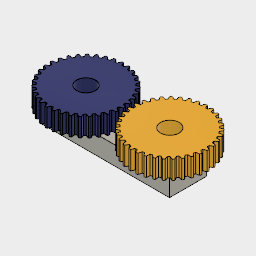
C04-W3-PE-01 (Autodesk Fusion 360 design; units mm, degrees)
Autodesk Fusion 360 part; units mm, degrees
sketch "Sketch1" plane through (0, 0, 0) normal (0, 1, 0) x (1, 0, 0) in component "Base Plate"
  line L0 (-87.5, 25) -> (87.5, 25)
  line L1 (87.5, 25) -> (87.5, -25)
  line L2 (87.5, -25) -> (-87.5, -25)
  line L3 (-87.5, -25) -> (-87.5, 25)
  line L4 (-87.5, 25) -> (87.5, -25) construction
  line L5 (87.5, 25) -> (-87.5, -25) construction
  circle A0 centre (-50, 0) radius 12.5
  circle A1 centre (50, 0) radius 12.5
  dimension "d1" = 175
  dimension "d2" = 50
  dimension "d3" = 25
  dimension "d4" = 50
  dimension "d5" = 50
  measures "d1" distance of L1.end L2.end
  measures "d2" distance of L0.end L1.end
  measures "d3" diameter of A1
  measures "d4" distance of origin A0.centre
  measures "d5" distance of origin A1.centre
extrude "Extrude1" add sketch "Sketch1" along normal blind 25 makes body 1 in component "Base Plate"
sketch "Sketch1 (2)" plane through (0, 25, 0) normal (0, 1, 0) x (-1, 0, 0) in component "Gear 1"
  circle A0 centre (-50, 0) radius 12.5
  circle A1 centre (50, 0) radius 12.5
  line L0 (87.5, 25) -> (-87.5, 25)
  line L1 (-87.5, 25) -> (-87.5, -25)
  line L2 (-87.5, -25) -> (87.5, -25)
  line L3 (87.5, -25) -> (87.5, 25)
  circle A2 centre (50, 0) radius 12.5
  circle A3 centre (50, 0) radius 47.5
  dimension "d19" = 95
  measures "d19" diameter of A3
extrude "Extrude1'" add sketch "Sketch1 (2)" along normal blind 25 separate body contours L0 L2 L3 A3 | L0 L2 L3 A3 makes body 2 in component "Gear 1"
sketch "Sketch2" plane through (0, 50, 0) normal (0, 1, 0) x (-1, 0, 0) in component "Gear 1"
  circle A0 centre (50, 0) radius 12.5
  circle A1 centre (50, 0) radius 47.5
  line L0 (0, 0) -> (-2, 0) construction
  arc A2 (-1.6663, 1.375) -> (-1.6663, -1.375) centre (1, 0) ccw
  line L1 (-1.6663, -1.375) -> (2.5901, -2.9242)
  line L2 (-1.6663, 1.375) -> (2.5901, 2.9242)
  dimension "d10" = 2
  dimension "d11" = 3
  dimension "d12" = 2.75
  dimension "d13" = 20
  dimension "d14" = 20
  measures "d10" distance of L0.start L0.end
  measures "d11" radius of A2
  measures "d12" distance of A2.end A2.start
  measures "d13" angle of L0 L1
  measures "d14" angle of L0 L2
extrude "Extrude2" add sketch "Sketch2" against normal blind 25 contours A1 A2 L1 L2 bodies 2 in component "Gear 1"
pattern_circular "C-Pattern1" count 35 over 360 about axis through (-50, 25, 0) along (0, 1, 0) of "Extrude2" in component "Gear 1"
sketch "Sketch1 (3)" plane through (0, 25, 0) normal (0, 1, 0) x (-1, 0, 0) in component "Gear 1 (1)"
  circle A0 centre (-50, 0) radius 12.5
  circle A1 centre (50, 0) radius 12.5
  line L0 (87.5, 25) -> (-87.5, 25)
  line L1 (-87.5, 25) -> (-87.5, -25)
  line L2 (-87.5, -25) -> (87.5, -25)
  line L3 (87.5, -25) -> (87.5, 25)
  circle A2 centre (50, 0) radius 12.5
  circle A3 centre (50, 0) radius 47.5
  dimension "d19_1" = 95
  measures "d19_1" diameter of A3
extrude "Extrude1''" add sketch "Sketch1 (3)" along normal blind 25 separate body contours L0 L2 L3 A3 | L0 L2 L3 A3 makes body 3 in component "Gear 1 (1)"
sketch "Sketch2 (2)" plane through (0, 50, 0) normal (0, 1, 0) x (-1, 0, 0) in component "Gear 1 (1)"
  circle A0 centre (50, 0) radius 12.5
  circle A1 centre (50, 0) radius 47.5
  line L0 (0, 0) -> (-2, 0) construction
  arc A2 (-1.6663, 1.375) -> (-1.6663, -1.375) centre (1, 0) ccw
  line L1 (-1.6663, -1.375) -> (2.5901, -2.9242)
  line L2 (-1.6663, 1.375) -> (2.5901, 2.9242)
  dimension "d10_1" = 2
  dimension "d11_1" = 3
  dimension "d12_1" = 2.75
  dimension "d13_1" = 20
  dimension "d14_1" = 20
  measures "d10_1" distance of L0.start L0.end
  measures "d11_1" radius of A2
  measures "d12_1" distance of A2.end A2.start
  measures "d13_1" angle of L0 L1
  measures "d14_1" angle of L0 L2
extrude "Extrude2'" add sketch "Sketch2 (2)" against normal blind 25 contours A1 A2 L1 L2 bodies 3 in component "Gear 1 (1)"
pattern_circular "C-Pattern1'" count 35 over 360 about axis through (-50, 25, 0) along (0, 1, 0) of "Extrude2'" in component "Gear 1 (1)"
component "Base Plate" placed x (1, 0, 0) y (0, 1, 0) z (0, 0, 1) at (0, 0, 0)
component "Gear 1" placed x (1, 0, 0) y (0, 1, 0) z (0, 0, 1) at (0, 0, 0)
component "Gear 1 (1)" placed x (1, 0, 0) y (0, 1, 0) z (0, 0, 1) at (106, 0, -7)
